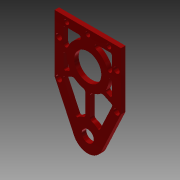
# Autodesk Inventor part: Swerve Wheel + Carriage Outline V1
Saved by Autodesk Inventor 2013 (Build 170138000, 138)
## iProperties
Created: 2013-04-01
Part Number: Swerve Wheel + Carriage Outline V1
Material: Generic
Document SubType Name: Sheet Metal
Designer: mvarma
Density: 1 g/cm^3
Sheet Metal Rule: Default
Author: mvarma
Autodesk Inventor part; units mm, degrees
ref_plane "YZ Plane" through (0, 0, 0) normal (1, 0, 0) x (0, 1, 0)
ref_plane "XZ Plane" through (0, 0, 0) normal (0, 1, 0) x (-1, 0, 0)
ref_plane "XY Plane" through (0, 0, 0) normal (0, 0, 1) x (1, 0, 0)
sketch "Sketch1" plane through (0, 0, 0) normal (0, 0, 1) x (1, 0, 0)
  circle A0 centre (0, 0) radius 38.1 construction
  circle A1 centre (0, 0) radius 41.275 construction
  line L0 (-7.3323, 0) -> (-3.6662, 6.35) construction
  line L1 (-3.6662, 6.35) -> (3.6662, 6.35) construction
  line L2 (3.6662, 6.35) -> (7.3323, 0) construction
  line L3 (7.3323, 0) -> (3.6662, -6.35) construction
  line L4 (3.6662, -6.35) -> (-3.6662, -6.35) construction
  line L5 (-3.6662, -6.35) -> (-7.3323, 0) construction
  circle A2 centre (0, 0) radius 6.35
  circle A3 centre (0, 0) radius 15.875 construction
  circle A4 centre (0, 0) radius 8.7313 construction
  circle A5 centre (0, 0) radius 15.875
  line L6 (34.925, 37.2364) -> (34.925, 97.5614)
  line L7 (34.925, 97.5614) -> (-34.925, 97.5614)
  line L8 (-34.925, 97.5614) -> (-34.925, 37.2364)
  line L9 (34.925, 37.2364) -> (-34.925, 37.2364) construction
  line L10 (34.925, 37.2364) -> (14.382, -6.7212)
  line L11 (-34.925, 37.2364) -> (-14.382, -6.7212)
  circle A6 centre (-30.353, 37.2364) radius 3.9624 construction
  line L12 (53.34, 97.5614) -> (-53.34, 97.5614) construction
  line L13 (-53.34, 97.5614) -> (-53.34, 107.0864) construction
  line L14 (-53.34, 107.0864) -> (53.34, 107.0864) construction
  line L15 (53.34, 107.0864) -> (53.34, 97.5614) construction
  circle A7 centre (-222.5199, 24.1494) radius 53.34 construction
  line L16 (-190.7699, 59.0744) -> (-254.2699, 59.0744) construction
  line L17 (-254.2699, 59.0744) -> (-254.2699, -10.7756) construction
  line L18 (-254.2699, -10.7756) -> (-190.7699, -10.7756) construction
  line L19 (-190.7699, -10.7756) -> (-190.7699, 59.0744) construction
  line L20 (-195.5324, 59.0744) -> (-195.5324, -10.7756) construction
  line L21 (-249.5074, 59.0744) -> (-249.5074, -10.7756) construction
  line L22 (-209.8199, 68.5994) -> (-235.2199, 68.5994) construction
  line L23 (-235.2199, 68.5994) -> (-235.2199, -20.3006) construction
  line L24 (-235.2199, -20.3006) -> (-209.8199, -20.3006) construction
  line L25 (-209.8199, -20.3006) -> (-209.8199, 68.5994) construction
  line L26 (34.925, 88.0364) -> (-34.925, 88.0364) construction
  circle A8 centre (30.353, 37.2364) radius 3.9624 construction
  circle A9 centre (30.353, 75.3364) radius 3.9624 construction
  circle A10 centre (-30.353, 75.3364) radius 3.9624 construction
  line L27 (34.925, 92.7989) -> (-34.925, 92.7989) construction
  circle A11 centre (0, 63.0333) radius 14.2875
  circle A12 centre (0, 63.0333) radius 15.875 construction
  line L28 (7.3323, 63.0333) -> (3.6662, 56.6833) construction
  line L29 (3.6662, 56.6833) -> (-3.6662, 56.6833) construction
  line L30 (-3.6662, 56.6833) -> (-7.3323, 63.0333) construction
  line L31 (-7.3323, 63.0333) -> (-3.6662, 69.3833) construction
  line L32 (-3.6662, 69.3833) -> (3.6662, 69.3833) construction
  line L33 (3.6662, 69.3833) -> (7.3323, 63.0333) construction
  point P0 (22.225, 92.7989)
  point P1 (0, 92.7989)
  point P2 (-22.225, 92.7989)
  dimension "d0" = 76.2
  dimension "d2" = 82.55
  dimension "d3" = 12.7
  dimension "d4" = 12.7
  dimension "d5" = 31.75
  dimension "d6" = 17.4625
  dimension "d7" = 31.75
  dimension "d8" = 69.85
  dimension "d9" = 34.925
  dimension "d10" = 37.2364
  dimension "d13" = 7.9248
  dimension "d14" = 9.525
  dimension "d15" = 106.68
  dimension "d16" = 53.34
  dimension "d17" = 106.68
  dimension "d18" = 69.85
  dimension "d19" = 34.925
  dimension "d20" = 63.5
  dimension "d21" = 31.75
  dimension "d22" = 4.7625
  dimension "d23" = 4.7625
  dimension "d24" = 25.4
  dimension "d25" = 14.2875
  dimension "d26" = 88.9
  dimension "d27" = 14.2875
  dimension "d28" = 44.45
  dimension "d29" = 4.572
  dimension "d30" = 9.525
  dimension "d31" = 0
  dimension "d32" = 7.9248
  dimension "d33" = 4.572
  dimension "d34" = 7.9248
  dimension "d35" = 7.9248
  dimension "d36" = 4.572
  dimension "d37" = 4.572
  dimension "d38" = 38.1
  dimension "d39" = 38.1
  dimension "d44" = 4.7625
  dimension "d45" = 34.925
  dimension "d46" = 12.7
  dimension "d47" = 12.7
  dimension "d48" = 28.575
  dimension "d52" = 31.75
  dimension "d53" = 12.7
  dimension "d54" = 25.0031
  dimension "d72" = 50.8
  dimension "d73" = 34.925
  constraints: 68 end point, 13 centre point, 13 coincident, 12 point on line, 10 perpendicular, 7 parallel, 5 horizontal, 2 point on circle, 2 tangent, 1 midpoint, 27 other
  measures "d0" diameter of A0
  measures "d2" diameter of A1
  measures "d3" distance between parallel lines of L4 L1
  measures "d4" diameter of A2
  measures "d5" diameter of A3
  measures "d6" diameter of A4
  measures "d7" diameter of A5
  measures "d8" distance between parallel lines of L8 L6
  measures "d9" distance from line of point (0, 0) L8
  measures "d10" distance from line of L9 point (0, 0)
  measures "d13" diameter of A6
  measures "d14" distance of L14.end L12.start
  measures "d15" distance of L13.end L14.end
  measures "d16" horizontal distance of L12.start point (0, 0)
  measures "d17" diameter of A7
  measures "d18" distance of L18.end L16.start
  measures "d19" distance from line of A7.centre L18
  measures "d20" distance of L17.end L18.end
  measures "d21" distance from line of L19 A7.centre
  measures "d22" distance between parallel lines of L17 L21
  measures "d23" distance between parallel lines of L19 L20
  measures "d24" distance between parallel lines of L23 L25
  measures "d25" distance between parallel lines of L20 L25
  measures "d26" distance of L22.end L23.end
  measures "d27" distance between parallel lines of L21 L23
  measures "d28" distance from line of A7.centre L24
  measures "d29" distance from line of L8 A6.centre
  measures "d30" distance between parallel lines of L7 L26
  measures "d31" distance between parallel lines of L7 L12
  measures "d32" diameter of A8
  measures "d33" distance from line of L6 A8.centre
  measures "d34" diameter of A9
  measures "d35" diameter of A10
  measures "d36" distance from line of L8 A10.centre
  measures "d37" distance from line of L6 A9.centre
  measures "d38" distance from line of L9 A10.centre
  measures "d39" distance from line of L9 A9.centre
  measures "d44" distance between parallel lines of L26 L27
  measures "d45" distance from line of L8 point (0, 92.799)
  measures "d46" distance from line of L8 point (-22.225, 92.799)
  measures "d47" distance from line of L6 point (22.225, 92.799)
  measures "d48" diameter of A11
  measures "d52" diameter of A12
  measures "d53" distance between parallel lines of L29 L32
  measures "d54" distance from line of L26 A12.centre
  measures "d72" distance between parallel lines of L9 L26
  measures "d73" distance from line of L8 A11.centre
extrude "Plate1" add sketch "Sketch1" along normal blind 4.7625 contours A2 | A5 | A5 L11 L8 L7 L6 L10 | A11
extrude "Cut1" cut sketch "Sketch1" along normal up to next contours A2 | A11
hole "Hole1" at (30.353, 75.3364, 0) at (30.353, 37.2364, 0) at (-30.353, 37.2364, 0) at (-30.353, 75.3364, 0) direction (0, 0, 1) diameter 6.35 end through all
hole "Hole2" at (22.225, 92.7989, 0) at (0, 92.7989, 0) at (-22.225, 92.7989, 0) direction (0, 0, 1) diameter 4.9784 end through all clearance for "Socket Head Cap Screw" size "#10" standard "Ansi Unified Screw Threads"
sketch "Sketch2" plane through (0, 0, 0) normal (0, 0, -1) x (-1, 0, 0)
  line L0 (-24.8576, 41.9413) -> (-16.7624, 45.7245)
  line L1 (24.8576, 41.9413) -> (16.7624, 45.7245)
  line L2 (-25.6237, 39.8309) -> (-12.8659, 12.5319)
  line L3 (12.8659, 12.5319) -> (25.6237, 39.8309)
  arc A0 (10.3888, 12.0037) -> (4.6302, 15.1848) centre (0, 0) ccw
  arc A1 (4.8617, 41.3465) -> (13.4909, 45.3712) centre (0, 63.0333) ccw
  arc A2 (-24.8576, 41.9413) -> (-25.6237, 39.8309) centre (-24.1855, 40.5031) ccw
  arc A3 (25.6237, 39.8309) -> (24.8576, 41.9413) centre (24.1855, 40.5031) ccw
  arc A4 (-12.8659, 12.5319) -> (-10.3888, 12.0037) centre (-11.4277, 13.2041) ccw
  arc A5 (-13.4909, 45.3712) -> (-4.8617, 41.3465) centre (0, 63.0333) ccw
  arc A6 (19.1632, 51.7761) -> (22.224, 62.8197) centre (0, 63.0333) ccw
  arc A7 (-13.4909, 45.3712) -> (-16.7624, 45.7245) centre (-15.4181, 42.8481) ccw
  arc A8 (16.7624, 45.7245) -> (13.4909, 45.3712) centre (15.4181, 42.8481) ccw
  line L4 (-25.6237, 39.8309) -> (-26.2958, 41.2691) construction
  line L5 (-24.8576, 41.9413) -> (-26.2958, 41.2691) construction
  line L6 (-23.1404, 48.0007) -> (-19.8598, 49.5338)
  line L7 (19.8598, 49.5338) -> (23.1404, 48.0007)
  line L8 (-25.4, 49.4389) -> (-25.4, 62.8197)
  line L9 (25.4, 49.4389) -> (25.4, 62.8197)
  line L10 (-25.4, 62.8197) -> (-22.224, 62.8197) construction
  line L11 (25.4, 62.8197) -> (22.224, 62.8197) construction
  arc A9 (-22.224, 62.8197) -> (-25.4, 62.8197) centre (-23.812, 62.8197) ccw
  arc A10 (25.4, 62.8197) -> (22.224, 62.8197) centre (23.812, 62.8197) ccw
  arc A11 (-25.4, 49.4389) -> (-23.1404, 48.0007) centre (-23.8125, 49.4389) ccw
  arc A12 (-19.8598, 49.5338) -> (-19.1632, 51.7761) centre (-20.532, 50.972) ccw
  arc A13 (19.1632, 51.7761) -> (19.8598, 49.5338) centre (20.532, 50.972) ccw
  arc A14 (23.1404, 48.0007) -> (25.4, 49.4389) centre (23.8125, 49.4389) ccw
  arc A15 (-22.224, 62.8197) -> (-19.1632, 51.7761) centre (0, 63.0333) ccw
  arc A16 (22.224, 62.8197) -> (20.7911, 70.8869) centre (0, 63.0333) ccw
  line L12 (-25.4, 62.8197) -> (-25.4, 86.4489)
  line L13 (-23.8125, 88.0364) -> (23.8125, 88.0364)
  line L14 (25.4, 86.4489) -> (25.4, 62.8197)
  arc A17 (-25.4, 71.7284) -> (-20.7911, 70.8869) centre (-23.0187, 71.7284) ccw
  arc A18 (-8.744, 83.4659) -> (-9.6808, 88.0364) centre (-9.6808, 85.6552) ccw
  arc A19 (9.6808, 88.0364) -> (8.744, 83.4659) centre (9.6808, 85.6552) ccw
  arc A20 (20.7911, 70.8869) -> (25.4, 71.7284) centre (23.0188, 71.7284) ccw
  arc A21 (-9.6808, 88.0364) -> (-8.744, 83.4659) centre (-9.6808, 85.6552) ccw
  arc A22 (-20.7911, 70.8869) -> (-25.4, 71.7284) centre (-23.0187, 71.7284) ccw
  arc A23 (8.744, 83.4659) -> (9.6808, 88.0364) centre (9.6808, 85.6552) ccw
  arc A24 (25.4, 71.7284) -> (20.7911, 70.8869) centre (23.0188, 71.7284) ccw
  arc A25 (20.7911, 70.8869) -> (8.744, 83.4659) centre (0, 63.0333) ccw
  arc A26 (8.744, 83.4659) -> (-8.744, 83.4659) centre (0, 63.0333) ccw
  arc A27 (-8.744, 83.4659) -> (-20.7911, 70.8869) centre (0, 63.0333) ccw
  arc A28 (-20.7911, 70.8869) -> (-22.224, 62.8197) centre (0, 63.0333) ccw
  arc A29 (-23.8125, 88.0364) -> (-25.4, 86.4489) centre (-23.8125, 86.4489) ccw
  arc A30 (25.4, 86.4489) -> (23.8125, 88.0364) centre (23.8125, 86.4489) ccw
  circle A31 centre (0, 92.7989) radius 2.4892 projected
  circle A32 centre (-22.225, 92.7989) radius 2.4892 projected
  circle A33 centre (22.225, 92.7989) radius 2.4892 projected
  circle A34 centre (30.353, 37.2364) radius 3.175 projected
  circle A35 centre (-30.353, 75.3364) radius 3.175 projected
  circle A36 centre (-30.353, 37.2364) radius 3.175 projected
  circle A37 centre (30.353, 75.3364) radius 3.175 projected
  circle A38 centre (0, 0) radius 6.35 projected
  circle A39 centre (0, 63.0333) radius 14.2875 projected
  arc A40 (-14.382, -6.7212) -> (14.382, -6.7212) centre (0, 0) ccw projected
  line L15 (34.925, 37.2364) -> (14.382, -6.7212) projected
  line L16 (34.925, 97.5614) -> (34.925, 37.2364) projected
  line L17 (-34.925, 97.5614) -> (34.925, 97.5614) projected
  line L18 (-34.925, 37.2364) -> (-34.925, 97.5614) projected
  line L19 (-14.382, -6.7212) -> (-34.925, 37.2364) projected
  line L20 (-26.2958, 41.2691) -> (-34.925, 37.2364) construction
  line L21 (24.3186, 42.1932) -> (34.925, 37.2364) construction
  arc A41 (10.3888, 12.0037) -> (12.8659, 12.5319) centre (11.4277, 13.2041) ccw
  arc A42 (-14.382, -6.7212) -> (14.382, -6.7212) centre (0, 0) ccw projected
  line L22 (0, 40.8083) -> (0, -15.875)
  line L23 (-2.3812, 38.2484) -> (-2.3812, 18.2217)
  line L24 (2.3813, 18.2217) -> (2.3813, 38.2484)
  arc A43 (-2.3812, 38.2484) -> (-4.8617, 41.3465) centre (-5.5562, 38.2484) ccw
  arc A44 (4.8617, 41.3465) -> (2.3813, 38.2484) centre (5.5563, 38.2484) ccw
  arc A45 (2.3813, 18.2217) -> (4.6302, 15.1848) centre (5.5563, 18.2217) ccw
  arc A46 (-4.6302, 15.1848) -> (-10.3888, 12.0037) centre (0, 0) ccw
  arc A47 (-4.6302, 15.1848) -> (-2.3812, 18.2217) centre (-5.5562, 18.2217) ccw
  point P0 (11.9129, 10.4928)
  point P1 (-25.4, 46.9447)
  point P2 (25.4, 46.9447)
  point P3 (-2.3812, 40.9362)
  point P4 (-2.3812, 15.6954)
  point P5 (2.3813, 15.6954)
  point P6 (2.3813, 40.9362)
  dimension "d79" = 1.5875
  dimension "d80" = 1.5875
  dimension "d81" = 3.175
  dimension "d84" = 4.7625
  dimension "d85" = 15.875
  dimension "d86" = 15.875
  dimension "d87" = 1.5875
  dimension "d89" = 4.7625
  dimension "d91" = 4.7625
  dimension "d92" = 1.5875
  dimension "d93" = 9.525
  dimension "d94" = 9.525
  dimension "d95" = 9.525
  dimension "d96" = 9.525
  dimension "d97" = 9.525
  dimension "d98" = 22.225
  dimension "d99" = 22.225
  dimension "d104" = 10.6064
  dimension "d107" = 15.875
  dimension "d108" = 1.5875
  dimension "d111" = 2.3813
  dimension "d112" = 4.7625
  dimension "d113" = 3.175
  dimension "d114" = 3.175
  dimension "d115" = 22.225
  constraints: 91 point on circle, 44 tangent, 40 end point, 37 centre point, 14 point on line, 11 equal radius, 9 perpendicular, 5 parallel, 3 coincident, 2 collinear, 2 midpoint, 1 vertical
  measures "d79" radius of A2
  measures "d80" radius of A4
  measures "d81" radius of A7
  measures "d84" distance between parallel lines of L6 L0
  measures "d85" distance of point (-25.4, 46.945) L8.end
  measures "d86" distance of point (25.4, 46.945) L9.end
  measures "d87" radius of A11
  measures "d89" distance between parallel lines of L1 L7
  measures "d91" diameter of A20
  measures "d92" radius of A29
  measures "d93" distance between parallel lines of L17 L13
  measures "d94" distance between parallel lines of L18 L12
  measures "d95" distance between parallel lines of L16 L14
  measures "d96" distance between parallel lines of L15 L3
  measures "d97" distance between parallel lines of L19 L2
  measures "d98" radius of A5
  measures "d99" radius of A15
  measures "d104" distance from line of L21.start L16
  measures "d107" radius of A0
  measures "d108" radius of A41
  measures "d111" distance between parallel lines of L22 L24
  measures "d112" distance between parallel lines of L23 L24
  measures "d113" radius of A43
  measures "d114" radius of A47
  measures "d115" radius of A1
extrude "Cut2" cut sketch "Sketch2" against normal blind 4.7625 contours L0 A7 A5 A43 L23 A47 A46 A4 L2 A2 | A3 L3 A41 A0 A45 L24 A44 A1 A8 L1 | A6 A10 L9 A14 L7 A13 | A24 A20 | A25 A23 L13 A30 L14 A24 | A19 A23 | A21 A18 | A27 A22 L12 A29 L13 A21 | A17 A22 | A15 A12 L6 A11 L8 A9
equation "\"d9\" = 0.5 * d8"
equation "\"d16\" = 0.5 * d15"
equation "\"d19\" = 0.5 * d18"
equation "\"d21\" = 0.5 * d20"
equation "\"d22\" = d23"
equation "\"d25\" = d27"
equation "\"d28\" = 0.5 * d26"
equation "\"d32\" = d13"
equation "\"d33\" = d29"
equation "\"d34\" = d32"
equation "\"d35\" = d13"
equation "\"d36\" = d29"
equation "\"d37\" = d29"
equation "\"d39\" = d38"
equation "\"d44\" = 0.5 * d30"
equation "\"d45\" = d42"
equation "\"d47\" = d46"
equation "\"d56\" = Thickness"
equation "\"d63\" = Thickness"
equation "\"d70\" = Thickness"
equation "\"d79\" = d80"
equation "\"BendRadius\" = Thickness"
equation "\"BendReliefWidth\" = Thickness"
equation "\"BendReliefDepth\" = 0.5 * Thickness"
equation "\"CornerReliefSize\" = 4 * Thickness"
equation "\"MinimumRemnant\" = 2 * Thickness"
equation "\"TransitionRadius\" = BendRadius"
equation "\"JacobiRadiusSize\" = Thickness"
equation "\"GapSize\" = Thickness"
equation "\"d55\" = BendRadius"
equation "\"Thickness\" = 4.7625"
equation "\"d42\" = 34.925"
body "Solid1"
